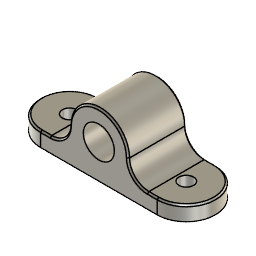
model (Autodesk Fusion 360 design; units mm, degrees)
part number: 2025-08-24-19-34-13-905
Autodesk Fusion 360 part; units mm, degrees
sketch "Sketch1" plane through (0, 0, 0) normal (0, 0, 1) x (1, 0, 0)
  line L0 (0.75, -0.375) -> (-0.75, -0.375)
  line L1 (-0.75, -0.375) -> (-0.75, 0.375) construction
  line L2 (-0.75, 0.375) -> (0.75, 0.375)
  line L3 (0.75, 0.375) -> (0.75, -0.375) construction
  line L4 (0.75, -0.375) -> (-0.75, 0.375) construction
  line L5 (-0.75, -0.375) -> (0.75, 0.375) construction
  arc A0 (-0.75, 0.375) -> (-0.75, -0.375) centre (-0.75, 0) ccw
  arc A1 (0.75, -0.375) -> (0.75, 0.375) centre (0.75, 0) ccw
  circle A2 centre (-0.75, 0) radius 0.094
  circle A3 centre (0.75, 0) radius 0.094
  dimension "d1" = 1.5
  dimension "d2" = 0.75
  dimension "d3" = 0.188
  constraint horizontal L0
  constraint perpendicular L0 L1
  constraint parallel L0 L2
  constraint parallel L1 L3
  constraint coincident L4 origin
  constraint coincident L5 origin
  constraint tangent L0 A0
  constraint tangent L2 A1
  constraint concentric A0 A2
  constraint concentric A1 A3
  constraint equal A2 A3
  measures "d1" distance of L1.end L2.end
  measures "d2" distance of L0 L2
  measures "d3" diameter of A2
extrude "Extrude1" add sketch "Sketch1" along normal blind 0.188
sketch "Sketch2" plane through (0, -0.375, 0) normal (0, -1, 0) x (1, 0, 0)
  line L0 (-0.75, 0) -> (0.75, 0)
  line L1 (0.75, 0) -> (0.75, 0.188)
  line L2 (0.75, 0.188) -> (-0.75, 0.188)
  line L3 (-0.75, 0.188) -> (-0.75, 0)
  line L4 (0, 0) -> (0, 0.837) construction
  line L5 (-0.375, 0.437) -> (-0.375, 0.188)
  line L6 (0.375, 0.437) -> (0.375, 0.188)
  arc A0 (0.375, 0.437) -> (-0.375, 0.437) centre (0, 0.437) ccw
  dimension "d6" = 0.75
  dimension "d7" = 0.437
  constraint coincident L4.start origin
  constraint perpendicular L0 L4
  constraint coincident L4 A0.centre
  constraint coincident L2 L5.end
  constraint perpendicular L2 L5
  constraint coincident L6.start A0
  constraint coincident L2 L6.end
  constraint perpendicular L2 L6
  constraint tangent L5 A0
  constraint tangent L6 A0
  constraint coincident L6 A0.start
  measures "d6" diameter of A0
  measures "d7" distance of L4.start A0.centre
extrude "Extrude2" add sketch "Sketch2" against normal up to surface (0.75 mm away) contours L2 L5 L6 A0
hole "Hole1" at (0, -0.375, 0.437) direction (0, 1, 0) diameter 0.4 end through all
fillet "Fillet1" radius 0.25 2 edges at (0.375, 0, 0.188) (-0.375, 0, 0.188)
chamfer "Chamfer1" distance 0.02 angle 45 12 edges at (-0.4486, -0.375, 0.2609) (-0.6875, -0.375, 0.188) (-1.125, 0, 0.188) (-0.6875, 0.375, 0.188) (-0.4486, 0.375, 0.2609) (0, 0.375, 0.812) (0.4486, 0.375, 0.2609) (0.6875, 0.375, 0.188) (1.125, 0, 0.188) (0.6875, -0.375, 0.188) (0.4486, -0.375, 0.2609) (0, -0.375, 0.812)
